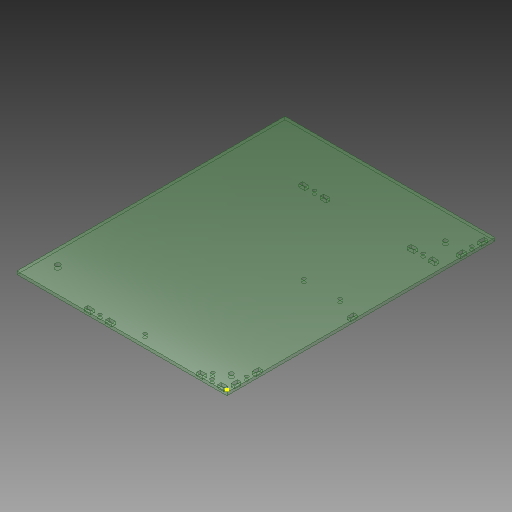
# Autodesk Inventor part: EE Base
Saved by Autodesk Inventor 2017 (Build 210142000, 142)
## iProperties
Created: 2016-07-27
Part Number: EE Base
Material: Polycarbonate, Green
Document SubType Name: Modeling
Designer: User
Density: 1.2 g/cm^3
Appearance: Polycarbonate - Clear(2)
Author: User
Autodesk Inventor part; units mm, degrees
(part 1 of 2)
ref_plane "YZ Plane" through (0, 0, 0) normal (1, 0, 0) x (0, 1, 0)
ref_plane "XZ Plane" through (0, 0, 0) normal (0, 1, 0) x (-1, 0, 0)
ref_plane "XY Plane" through (0, 0, 0) normal (0, 0, 1) x (1, 0, 0)
sketch "Sketch1" plane through (0, 0, 0) normal (0, 1, 0) x (-1, 0, 0)
  line L0 (-2.2365, 1.8101) -> (-2.2365, -264.9073)
  line L1 (-2.2365, -264.9073) -> (206.7635, -264.9073)
  line L2 (206.7635, -264.9073) -> (206.7635, 1.8101)
  line L3 (206.7635, 1.8101) -> (-2.2365, 1.8101)
  line L4 (58.9938, -133.7673) -> (58.8239, -133.3573)
  line L5 (58.8239, -133.3573) -> (58.5538, -133.0053)
  line L6 (58.5538, -133.0053) -> (58.2017, -132.7351)
  line L7 (58.2017, -132.7351) -> (57.7917, -132.5653)
  line L8 (57.7917, -132.5653) -> (57.3517, -132.5073)
  line L9 (57.3517, -132.5073) -> (56.9117, -132.5653)
  line L10 (56.9117, -132.5653) -> (56.5017, -132.7351)
  line L11 (56.5017, -132.7351) -> (56.1496, -133.0053)
  line L12 (56.1496, -133.0053) -> (55.8794, -133.3573)
  line L13 (55.8794, -133.3573) -> (55.7096, -133.7673)
  line L14 (55.7096, -133.7673) -> (55.6517, -134.2073)
  line L15 (55.6517, -134.2073) -> (55.7096, -134.6473)
  line L16 (55.7096, -134.6473) -> (55.8794, -135.0573)
  line L17 (55.8794, -135.0573) -> (56.1496, -135.4094)
  line L18 (56.1496, -135.4094) -> (56.5017, -135.6796)
  line L19 (56.5017, -135.6796) -> (56.9117, -135.8494)
  line L20 (56.9117, -135.8494) -> (57.3517, -135.9073)
  line L21 (57.3517, -135.9073) -> (57.7917, -135.8494)
  line L22 (57.7917, -135.8494) -> (58.2017, -135.6796)
  line L23 (58.2017, -135.6796) -> (58.5538, -135.4094)
  line L24 (58.5538, -135.4094) -> (58.8239, -135.0573)
  line L25 (58.8239, -135.0573) -> (58.9938, -134.6473)
  line L26 (58.9938, -134.6473) -> (59.0517, -134.2073)
  line L27 (59.0517, -134.2073) -> (58.9938, -133.7673)
  line L28 (21.4352, -215.2075) -> (21.3112, -214.8261)
  line L29 (21.3112, -214.8261) -> (21.0963, -214.4874)
  line L30 (21.0963, -214.4874) -> (20.8039, -214.2129)
  line L31 (20.8039, -214.2129) -> (20.4525, -214.0196)
  line L32 (20.4525, -214.0196) -> (20.064, -213.9199)
  line L33 (20.064, -213.9199) -> (19.663, -213.9199)
  line L34 (19.663, -213.9199) -> (19.2745, -214.0196)
  line L35 (19.2745, -214.0196) -> (18.923, -214.2129)
  line L36 (18.923, -214.2129) -> (18.6307, -214.4874)
  line L37 (18.6307, -214.4874) -> (18.4157, -214.8261)
  line L38 (18.4157, -214.8261) -> (18.2918, -215.2075)
  line L39 (18.2918, -215.2075) -> (18.2666, -215.6077)
  line L40 (18.2666, -215.6077) -> (18.3418, -216.0017)
  line L41 (18.3418, -216.0017) -> (18.5126, -216.3646)
  line L42 (18.5126, -216.3646) -> (18.7682, -216.6737)
  line L43 (18.7682, -216.6737) -> (19.0927, -216.9094)
  line L44 (19.0927, -216.9094) -> (19.4656, -217.057)
  line L45 (19.4656, -217.057) -> (19.8635, -217.1073)
  line L46 (19.8635, -217.1073) -> (20.2614, -217.057)
  line L47 (20.2614, -217.057) -> (20.6343, -216.9094)
  line L48 (20.6343, -216.9094) -> (20.9587, -216.6737)
  line L49 (20.9587, -216.6737) -> (21.2144, -216.3646)
  line L50 (21.2144, -216.3646) -> (21.3852, -216.0017)
  line L51 (21.3852, -216.0017) -> (21.42, -215.8311)
  line L52 (21.42, -215.8311) -> (21.4247, -215.8041)
  line L53 (21.4247, -215.8041) -> (21.4604, -215.6077)
  line L54 (21.4604, -215.6077) -> (21.4352, -215.2075)
  line L55 (13.929, -15.8348) -> (13.7092, -15.3042)
  line L56 (13.7092, -15.3042) -> (13.3596, -14.8486)
  line L57 (13.3596, -14.8486) -> (12.904, -14.499)
  line L58 (12.904, -14.499) -> (12.3734, -14.2792)
  line L59 (12.3734, -14.2792) -> (11.804, -14.2042)
  line L60 (11.804, -14.2042) -> (11.2346, -14.2792)
  line L61 (11.2346, -14.2792) -> (10.704, -14.499)
  line L62 (10.704, -14.499) -> (10.2483, -14.8486)
  line L63 (10.2483, -14.8486) -> (9.8987, -15.3042)
  line L64 (9.8987, -15.3042) -> (9.679, -15.8348)
  line L65 (9.679, -15.8348) -> (9.604, -16.4042)
  line L66 (9.604, -16.4042) -> (9.679, -16.9736)
  line L67 (9.679, -16.9736) -> (9.8987, -17.5042)
  line L68 (9.8987, -17.5042) -> (10.2483, -17.9599)
  line L69 (10.2483, -17.9599) -> (10.704, -18.3095)
  line L70 (10.704, -18.3095) -> (11.2346, -18.5293)
  line L71 (11.2346, -18.5293) -> (11.804, -18.6042)
  line L72 (11.804, -18.6042) -> (12.3734, -18.5293)
  line L73 (12.3734, -18.5293) -> (12.904, -18.3095)
  line L74 (12.904, -18.3095) -> (13.3596, -17.9599)
  line L75 (13.3596, -17.9599) -> (13.7092, -17.5042)
  line L76 (13.7092, -17.5042) -> (13.929, -16.9736)
  line L77 (13.929, -16.9736) -> (14.004, -16.4042)
  line L78 (14.004, -16.4042) -> (13.929, -15.8348)
  line L79 (2.7635, -0.1899) -> (2.7635, -3.7899)
  line L80 (2.7635, -3.7899) -> (8.9635, -3.7899)
  line L81 (8.9635, -3.7899) -> (8.9635, -0.1899)
  line L82 (8.9635, -0.1899) -> (2.7635, -0.1899)
  line L83 (3.1511, -245.3183) -> (2.9579, -244.9669)
  line L84 (2.9579, -244.9669) -> (2.6834, -244.6745)
  line L85 (2.6834, -244.6745) -> (2.3447, -244.4596)
  line L86 (2.3447, -244.4596) -> (1.9633, -244.3357)
  line L87 (1.9633, -244.3357) -> (1.5631, -244.3105)
  line L88 (1.5631, -244.3105) -> (1.1691, -244.3856)
  line L89 (1.1691, -244.3856) -> (0.8062, -244.5564)
  line L90 (0.8062, -244.5564) -> (0.4971, -244.812)
  line L91 (0.4971, -244.812) -> (0.2614, -245.1365)
  line L92 (0.2614, -245.1365) -> (0.1138, -245.5095)
  line L93 (0.1138, -245.5095) -> (0.0635, -245.9073)
  line L94 (0.0635, -245.9073) -> (0.1138, -246.3052)
  line L95 (0.1138, -246.3052) -> (0.2614, -246.6782)
  line L96 (0.2614, -246.6782) -> (0.4971, -247.0026)
  line L97 (0.4971, -247.0026) -> (0.8062, -247.2583)
  line L98 (0.8062, -247.2583) -> (1.1691, -247.429)
  line L99 (1.1691, -247.429) -> (1.5631, -247.5042)
  line L100 (1.5631, -247.5042) -> (1.9633, -247.479)
  line L101 (1.9633, -247.479) -> (2.3447, -247.3551)
  line L102 (2.3447, -247.3551) -> (2.6834, -247.1402)
  line L103 (2.6834, -247.1402) -> (2.9579, -246.8478)
  line L104 (2.9579, -246.8478) -> (3.1511, -246.4963)
  line L105 (3.1511, -246.4963) -> (3.2509, -246.1079)
  line L106 (3.2509, -246.1079) -> (3.2509, -245.7068)
  line L107 (3.2509, -245.7068) -> (3.1511, -245.3183)
  line L108 (-0.2365, -232.2073) -> (-0.2365, -238.4073)
  line L109 (-0.2365, -238.4073) -> (3.3635, -238.4073)
  line L110 (3.3635, -238.4073) -> (3.3635, -232.2073)
  line L111 (3.3635, -232.2073) -> (-0.2365, -232.2073)
  line L112 (-0.2365, -123.4758) -> (-0.2365, -129.7758)
  line L113 (-0.2365, -129.7758) -> (3.3635, -129.7758)
  line L114 (3.3635, -129.7758) -> (3.3635, -123.4758)
  line L115 (3.3635, -123.4758) -> (-0.2365, -123.4758)
  line L116 (3.1511, -21.0183) -> (2.9579, -20.6669)
  line L117 (2.9579, -20.6669) -> (2.6834, -20.3745)
  line L118 (2.6834, -20.3745) -> (2.3447, -20.1596)
  line L119 (2.3447, -20.1596) -> (1.9633, -20.0357)
  line L120 (1.9633, -20.0357) -> (1.5631, -20.0105)
  line L121 (1.5631, -20.0105) -> (1.1691, -20.0856)
  line L122 (1.1691, -20.0856) -> (0.8062, -20.2564)
  line L123 (0.8062, -20.2564) -> (0.4971, -20.5121)
  line L124 (0.4971, -20.5121) -> (0.2614, -20.8365)
  line L125 (0.2614, -20.8365) -> (0.1138, -21.2095)
  line L126 (0.1138, -21.2095) -> (0.0635, -21.6073)
  line L127 (0.0635, -21.6073) -> (0.1138, -22.0052)
  line L128 (0.1138, -22.0052) -> (0.2614, -22.3781)
  line L129 (0.2614, -22.3781) -> (0.4971, -22.7026)
  line L130 (0.4971, -22.7026) -> (0.8062, -22.9582)
  line L131 (0.8062, -22.9582) -> (1.1691, -23.129)
  line L132 (1.1691, -23.129) -> (1.5631, -23.2042)
  line L133 (1.5631, -23.2042) -> (1.9633, -23.179)
  line L134 (1.9633, -23.179) -> (2.3447, -23.0551)
  line L135 (2.3447, -23.0551) -> (2.6834, -22.8401)
  line L136 (2.6834, -22.8401) -> (2.9579, -22.5478)
  line L137 (2.9579, -22.5478) -> (3.1511, -22.1963)
  line L138 (3.1511, -22.1963) -> (3.2509, -21.8078)
  line L139 (3.2509, -21.8078) -> (3.2509, -21.4068)
  line L140 (3.2509, -21.4068) -> (3.1511, -21.0183)
  line L141 (6.1635, -213.6073) -> (6.1635, -217.2073)
  line L142 (6.1635, -217.2073) -> (12.3635, -217.2073)
  line L143 (12.3635, -217.2073) -> (12.3635, -213.6073)
  line L144 (12.3635, -213.6073) -> (6.1635, -213.6073)
  line L145 (-0.2365, -7.9073) -> (-0.2365, -14.1073)
  line L146 (-0.2365, -14.1073) -> (3.3635, -14.1073)
  line L147 (3.3635, -14.1073) -> (3.3635, -7.9073)
  line L148 (3.3635, -7.9073) -> (-0.2365, -7.9073)
  line L149 (-0.2365, -253.4073) -> (-0.2365, -259.6074)
  line L150 (-0.2365, -259.6074) -> (3.3635, -259.6074)
  line L151 (3.3635, -259.6074) -> (3.3635, -253.4073)
  line L152 (3.3635, -253.4073) -> (-0.2365, -253.4073)
  line L153 (-0.2365, -29.1073) -> (-0.2365, -35.3073)
  line L154 (-0.2365, -35.3073) -> (3.3635, -35.3073)
  line L155 (3.3635, -35.3073) -> (3.3635, -29.1073)
  line L156 (3.3635, -29.1073) -> (-0.2365, -29.1073)
  line L157 (18.0352, -1.7901) -> (17.9112, -1.4087)
  line L158 (17.9112, -1.4087) -> (17.6963, -1.07)
  line L159 (17.6963, -1.07) -> (17.4039, -0.7955)
  line L160 (17.4039, -0.7955) -> (17.0525, -0.6023)
  line L161 (17.0525, -0.6023) -> (16.664, -0.5025)
  line L162 (16.664, -0.5025) -> (16.263, -0.5025)
  line L163 (16.263, -0.5025) -> (15.8745, -0.6023)
  line L164 (15.8745, -0.6023) -> (15.523, -0.7955)
  line L165 (15.523, -0.7955) -> (15.2307, -1.07)
  line L166 (15.2307, -1.07) -> (15.0158, -1.4087)
  line L167 (15.0158, -1.4087) -> (14.8918, -1.7901)
  line L168 (14.8918, -1.7901) -> (14.8667, -2.1903)
  line L169 (14.8667, -2.1903) -> (14.9418, -2.5843)
  line L170 (14.9418, -2.5843) -> (15.1126, -2.9472)
  line L171 (15.1126, -2.9472) -> (15.3682, -3.2563)
  line L172 (15.3682, -3.2563) -> (15.6927, -3.492)
  line L173 (15.6927, -3.492) -> (16.0656, -3.6396)
  line L174 (16.0656, -3.6396) -> (16.4635, -3.6899)
  line L175 (16.4635, -3.6899) -> (16.8614, -3.6396)
  line L176 (16.8614, -3.6396) -> (17.2343, -3.492)
  line L177 (17.2343, -3.492) -> (17.5587, -3.2563)
  line L178 (17.5587, -3.2563) -> (17.8144, -2.9472)
  line L179 (17.8144, -2.9472) -> (17.9852, -2.5843)
  line L180 (17.9852, -2.5843) -> (18.0604, -2.1903)
  line L181 (18.0604, -2.1903) -> (18.0352, -1.7901)
  line L182 (23.4056, -7.4674) -> (23.2357, -7.0573)
  line L183 (23.2357, -7.0573) -> (22.9656, -6.7052)
  line L184 (22.9656, -6.7052) -> (22.6135, -6.4351)
  line L185 (22.6135, -6.4351) -> (22.2035, -6.2653)
  line L186 (22.2035, -6.2653) -> (21.7635, -6.2073)
  line L187 (21.7635, -6.2073) -> (21.3235, -6.2653)
  line L188 (21.3235, -6.2653) -> (20.9135, -6.4351)
  line L189 (20.9135, -6.4351) -> (20.5614, -6.7052)
  line L190 (20.5614, -6.7052) -> (20.2912, -7.0573)
  line L191 (20.2912, -7.0573) -> (20.1214, -7.4674)
  line L192 (20.1214, -7.4674) -> (20.0635, -7.9073)
  line L193 (20.0635, -7.9073) -> (20.1214, -8.3473)
  line L194 (20.1214, -8.3473) -> (20.2912, -8.7573)
  line L195 (20.2912, -8.7573) -> (20.5614, -9.1094)
  line L196 (20.5614, -9.1094) -> (20.9135, -9.3796)
  line L197 (20.9135, -9.3796) -> (21.3235, -9.5494)
  line L198 (21.3235, -9.5494) -> (21.7635, -9.6073)
  line L199 (21.7635, -9.6073) -> (22.2035, -9.5494)
  line L200 (22.2035, -9.5494) -> (22.6135, -9.3796)
  line L201 (22.6135, -9.3796) -> (22.9656, -9.1094)
  line L202 (22.9656, -9.1094) -> (23.2357, -8.7573)
  line L203 (23.2357, -8.7573) -> (23.4056, -8.3473)
  line L204 (23.4056, -8.3473) -> (23.4635, -7.9073)
  line L205 (23.4635, -7.9073) -> (23.4056, -7.4674)
  line L206 (23.7088, -134.5768) -> (23.539, -134.1668)
  line L207 (23.539, -134.1668) -> (23.2688, -133.8147)
  line L208 (23.2688, -133.8147) -> (22.9168, -133.5446)
  line L209 (22.9168, -133.5446) -> (22.5068, -133.3747)
  line L210 (22.5068, -133.3747) -> (22.0667, -133.3168)
  line L211 (22.0667, -133.3168) -> (21.6268, -133.3747)
  line L212 (21.6268, -133.3747) -> (21.2168, -133.5446)
  line L213 (21.2168, -133.5446) -> (20.8647, -133.8147)
  line L214 (20.8647, -133.8147) -> (20.5945, -134.1668)
  line L215 (20.5945, -134.1668) -> (20.4247, -134.5768)
  line L216 (20.4247, -134.5768) -> (20.3668, -135.0168)
  line L217 (20.3668, -135.0168) -> (20.4247, -135.4568)
  line L218 (20.4247, -135.4568) -> (20.5945, -135.8668)
  line L219 (20.5945, -135.8668) -> (20.8647, -136.2189)
  line L220 (20.8647, -136.2189) -> (21.2168, -136.489)
  line L221 (21.2168, -136.489) -> (21.6268, -136.6589)
  line L222 (21.6268, -136.6589) -> (22.0667, -136.7168)
  line L223 (22.0667, -136.7168) -> (22.5068, -136.6589)
  line L224 (22.5068, -136.6589) -> (22.9168, -136.489)
  line L225 (22.9168, -136.489) -> (23.2688, -136.2189)
  line L226 (23.2688, -136.2189) -> (23.539, -135.8668)
  line L227 (23.539, -135.8668) -> (23.7088, -135.4568)
  line L228 (23.7088, -135.4568) -> (23.7667, -135.0168)
  line L229 (23.7667, -135.0168) -> (23.7088, -134.5768)
  line L230 (27.3634, -213.6073) -> (27.3634, -217.2073)
  line L231 (27.3634, -217.2073) -> (33.5635, -217.2073)
  line L232 (33.5635, -217.2073) -> (33.5635, -213.6073)
  line L233 (33.5635, -213.6073) -> (27.3634, -213.6073)
  line L234 (23.9635, -0.1899) -> (23.9635, -3.7899)
  line L235 (23.9635, -3.7899) -> (30.1635, -3.7899)
  line L236 (30.1635, -3.7899) -> (30.1635, -0.1899)
  line L237 (30.1635, -0.1899) -> (23.9635, -0.1899)
  line L238 (90.6056, -7.461) -> (90.4357, -7.051)
  line L239 (90.4357, -7.051) -> (90.1656, -6.6989)
  line L240 (90.1656, -6.6989) -> (89.8135, -6.4288)
  line L241 (89.8135, -6.4288) -> (89.4035, -6.2589)
  line L242 (89.4035, -6.2589) -> (88.9635, -6.201)
  line L243 (88.9635, -6.201) -> (88.5235, -6.2589)
  line L244 (88.5235, -6.2589) -> (88.1135, -6.4288)
  line L245 (88.1135, -6.4288) -> (87.7614, -6.6989)
  line L246 (87.7614, -6.6989) -> (87.4913, -7.051)
  line L247 (87.4913, -7.051) -> (87.3214, -7.461)
  line L248 (87.3214, -7.461) -> (87.2635, -7.901)
  line L249 (87.2635, -7.901) -> (87.3214, -8.341)
  line L250 (87.3214, -8.341) -> (87.4913, -8.751)
  line L251 (87.4913, -8.751) -> (87.7614, -9.1031)
  line L252 (87.7614, -9.1031) -> (88.1135, -9.3733)
  line L253 (88.1135, -9.3733) -> (88.5235, -9.5431)
  line L254 (88.5235, -9.5431) -> (88.9635, -9.601)
  line L255 (88.9635, -9.601) -> (89.4035, -9.5431)
  line L256 (89.4035, -9.5431) -> (89.8135, -9.3733)
  line L257 (89.8135, -9.3733) -> (90.1656, -9.1031)
  line L258 (90.1656, -9.1031) -> (90.4357, -8.751)
  line L259 (90.4357, -8.751) -> (90.6056, -8.341)
  line L260 (90.6056, -8.341) -> (90.6635, -7.901)
  line L261 (90.6635, -7.901) -> (90.6056, -7.461)
  line L262 (114.3635, -213.6073) -> (114.3635, -217.2073)
  line L263 (114.3635, -217.2073) -> (120.5635, -217.2073)
  line L264 (120.5635, -217.2073) -> (120.5635, -213.6073)
  line L265 (120.5635, -213.6073) -> (114.3635, -213.6073)
  line L266 (129.6352, -215.2075) -> (129.5112, -214.8261)
  line L267 (129.5112, -214.8261) -> (129.2963, -214.4874)
  line L268 (129.2963, -214.4874) -> (129.0039, -214.2129)
  line L269 (129.0039, -214.2129) -> (128.6525, -214.0196)
  line L270 (128.6525, -214.0196) -> (128.264, -213.9199)
  line L271 (128.264, -213.9199) -> (127.863, -213.9199)
  line L272 (127.863, -213.9199) -> (127.4745, -214.0196)
  line L273 (127.4745, -214.0196) -> (127.123, -214.2129)
  line L274 (127.123, -214.2129) -> (126.8307, -214.4874)
  line L275 (126.8307, -214.4874) -> (126.6158, -214.8261)
  line L276 (126.6158, -214.8261) -> (126.4918, -215.2075)
  line L277 (126.4918, -215.2075) -> (126.4666, -215.6077)
  line L278 (126.4666, -215.6077) -> (126.5418, -216.0017)
  line L279 (126.5418, -216.0017) -> (126.7125, -216.3646)
  line L280 (126.7125, -216.3646) -> (126.9682, -216.6737)
  line L281 (126.9682, -216.6737) -> (127.2927, -216.9094)
  line L282 (127.2927, -216.9094) -> (127.6656, -217.057)
  line L283 (127.6656, -217.057) -> (128.0635, -217.1073)
  line L284 (128.0635, -217.1073) -> (128.4614, -217.057)
  line L285 (128.4614, -217.057) -> (128.8343, -216.9094)
  line L286 (128.8343, -216.9094) -> (129.1588, -216.6737)
  line L287 (129.1588, -216.6737) -> (129.4144, -216.3646)
  line L288 (129.4144, -216.3646) -> (129.5852, -216.0017)
  line L289 (129.5852, -216.0017) -> (129.6603, -215.6077)
  line L290 (129.6603, -215.6077) -> (129.6352, -215.2075)
  line L291 (194.4204, -23.2582) -> (194.1699, -22.6533)
  line L292 (194.1699, -22.6533) -> (193.7713, -22.1339)
  line L293 (193.7713, -22.1339) -> (193.2519, -21.7353)
  line L294 (193.2519, -21.7353) -> (192.647, -21.4848)
  line L295 (192.647, -21.4848) -> (191.9979, -21.3993)
  line L296 (191.9979, -21.3993) -> (191.3488, -21.4848)
  line L297 (191.3488, -21.4848) -> (190.7439, -21.7353)
  line L298 (190.7439, -21.7353) -> (190.2245, -22.1339)
  line L299 (190.2245, -22.1339) -> (189.8259, -22.6533)
  line L300 (189.8259, -22.6533) -> (189.5754, -23.2582)
  line L301 (189.5754, -23.2582) -> (189.4899, -23.9073)
  line L302 (189.4899, -23.9073) -> (189.5754, -24.5564)
  line L303 (189.5754, -24.5564) -> (189.8259, -25.1613)
  line L304 (189.8259, -25.1613) -> (190.2245, -25.6807)
  line L305 (190.2245, -25.6807) -> (190.7439, -26.0793)
  line L306 (190.7439, -26.0793) -> (191.3488, -26.3299)
  line L307 (191.3488, -26.3299) -> (191.9979, -26.4153)
  line L308 (191.9979, -26.4153) -> (192.647, -26.3299)
  line L309 (192.647, -26.3299) -> (193.2519, -26.0793)
  line L310 (193.2519, -26.0793) -> (193.7713, -25.6807)
  line L311 (193.7713, -25.6807) -> (194.1699, -25.1613)
  line L312 (194.1699, -25.1613) -> (194.4204, -24.5564)
  line L313 (194.4204, -24.5564) -> (194.5059, -23.9073)
  line L314 (194.5059, -23.9073) -> (194.4204, -23.2582)
  line L315 (135.5635, -213.6073) -> (135.5635, -217.2073)
  line L316 (135.5635, -217.2073) -> (141.7635, -217.2073)
  line L317 (141.7635, -217.2073) -> (141.7635, -213.6073)
  line L318 (141.7635, -213.6073) -> (135.5635, -213.6073)
  line L319 (135.5635, -0.1899) -> (135.5635, -3.7899)
  line L320 (135.5635, -3.7899) -> (141.7635, -3.7899)
  line L321 (141.7635, -3.7899) -> (141.7635, -0.1899)
  line L322 (141.7635, -0.1899) -> (135.5635, -0.1899)
  line L323 (114.3635, -0.1899) -> (114.3635, -3.7899)
  line L324 (114.3635, -3.7899) -> (120.5635, -3.7899)
  line L325 (120.5635, -3.7899) -> (120.5635, -0.1899)
  line L326 (120.5635, -0.1899) -> (114.3635, -0.1899)
  line L327 (129.6352, -1.7901) -> (129.5112, -1.4087)
  line L328 (129.5112, -1.4087) -> (129.2963, -1.07)
  line L329 (129.2963, -1.07) -> (129.0039, -0.7955)
  line L330 (129.0039, -0.7955) -> (128.6525, -0.6023)
  line L331 (128.6525, -0.6023) -> (128.264, -0.5025)
  line L332 (128.264, -0.5025) -> (127.863, -0.5025)
  line L333 (127.863, -0.5025) -> (127.4745, -0.6023)
  line L334 (127.4745, -0.6023) -> (127.123, -0.7955)
  line L335 (127.123, -0.7955) -> (126.8307, -1.07)
  line L336 (126.8307, -1.07) -> (126.6158, -1.4087)
  line L337 (126.6158, -1.4087) -> (126.4918, -1.7901)
  line L338 (126.4918, -1.7901) -> (126.4666, -2.1903)
  line L339 (126.4666, -2.1903) -> (126.5418, -2.5843)
  line L340 (126.5418, -2.5843) -> (126.7125, -2.9472)
  line L341 (126.7125, -2.9472) -> (126.9682, -3.2563)
  line L342 (126.9682, -3.2563) -> (127.2927, -3.492)
  line L343 (127.2927, -3.492) -> (127.6656, -3.6396)
  line L344 (127.6656, -3.6396) -> (128.0635, -3.6899)
  line L345 (128.0635, -3.6899) -> (128.4614, -3.6396)
  line L346 (128.4614, -3.6396) -> (128.8343, -3.492)
  line L347 (128.8343, -3.492) -> (129.1588, -3.2563)
  line L348 (129.1588, -3.2563) -> (129.4144, -2.9472)
  line L349 (129.4144, -2.9472) -> (129.5852, -2.5843)
  line L350 (129.5852, -2.5843) -> (129.6603, -2.1903)
  line L351 (129.6603, -2.1903) -> (129.6352, -1.7901)
  line L352 (21.8831, -237.0851) -> (21.685, -236.5461)
  line L353 (21.685, -236.5461) -> (21.354, -236.0767)
  line L354 (21.354, -236.0767) -> (20.9129, -235.7089)
  line L355 (20.9129, -235.7089) -> (20.3916, -235.4679)
  line L356 (20.3916, -235.4679) -> (19.8257, -235.37)
  line L357 (19.8257, -235.37) -> (19.2537, -235.4219)
  line L358 (19.2537, -235.4219) -> (18.7147, -235.6201)
  line L359 (18.7147, -235.6201) -> (18.2453, -235.951)
  line L360 (18.2453, -235.951) -> (17.8776, -236.3922)
  line L361 (17.8776, -236.3922) -> (17.6365, -236.9134)
  line L362 (17.6365, -236.9134) -> (17.5386, -237.4793)
  line L363 (17.5386, -237.4793) -> (17.5905, -238.0513)
  line L364 (17.5905, -238.0513) -> (17.7887, -238.5903)
  line L365 (17.7887, -238.5903) -> (18.1196, -239.0597)
  line L366 (18.1196, -239.0597) -> (18.5608, -239.4274)
  line L367 (18.5608, -239.4274) -> (19.0821, -239.6685)
  line L368 (19.0821, -239.6685) -> (19.648, -239.7664)
  line L369 (19.648, -239.7664) -> (20.22, -239.7145)
  line L370 (20.22, -239.7145) -> (20.759, -239.5163)
  line L371 (20.759, -239.5163) -> (21.2284, -239.1854)
  line L372 (21.2284, -239.1854) -> (21.5961, -238.7443)
  line L373 (21.5961, -238.7443) -> (21.8371, -238.223)
  line L374 (21.8371, -238.223) -> (21.9351, -237.6571)
  line L375 (21.9351, -237.6571) -> (21.8831, -237.0851)
  point P0 (0, 0)
  constraints: 752 end point
extrude "Extrusion1" add sketch "Sketch1" along normal blind 3
sketch "Sketch2" plane through (0, 3, 0) normal (0, 1, 0) x (1, 0, 0)
  line L0 (0.2365, 123.4758) -> (-3.3635, 123.4758) projected
  line L1 (-3.3635, 123.4758) -> (-3.3635, 129.7758) projected
  line L2 (-3.3635, 129.7758) -> (0.2365, 129.7758) projected
  line L3 (0.2365, 129.7758) -> (0.2365, 123.4758) projected
  line L4 (-23.9635, 0.1899) -> (-30.1635, 0.1899) projected
  line L5 (-30.1635, 0.1899) -> (-30.1635, 3.7899) projected
  line L6 (-30.1635, 3.7899) -> (-23.9635, 3.7899) projected
  line L7 (-23.9635, 3.7899) -> (-23.9635, 0.1899) projected
  line L8 (-27.3634, 213.6073) -> (-33.5635, 213.6073) projected
  line L9 (-33.5635, 213.6073) -> (-33.5635, 217.2073) projected
  line L10 (-33.5635, 217.2073) -> (-27.3634, 217.2073) projected
  line L11 (-27.3634, 217.2073) -> (-27.3634, 213.6073) projected
  line L12 (-135.5635, 0.1899) -> (-141.7635, 0.1899) projected
  line L13 (-141.7635, 0.1899) -> (-141.7635, 3.7899) projected
  line L14 (-141.7635, 3.7899) -> (-135.5635, 3.7899) projected
  line L15 (-135.5635, 3.7899) -> (-135.5635, 0.1899) projected
  line L16 (-135.5635, 213.6073) -> (-141.7635, 213.6073) projected
  line L17 (-141.7635, 213.6073) -> (-141.7635, 217.2073) projected
  line L18 (-141.7635, 217.2073) -> (-135.5635, 217.2073) projected
  line L19 (-135.5635, 217.2073) -> (-135.5635, 213.6073) projected
  line L20 (0.2365, 29.1073) -> (-3.3635, 29.1073) projected
  line L21 (-3.3635, 29.1073) -> (-3.3635, 35.3073) projected
  line L22 (-3.3635, 35.3073) -> (0.2365, 35.3073) projected
  line L23 (0.2365, 35.3073) -> (0.2365, 29.1073) projected
  line L24 (0.2365, 253.4073) -> (-3.3635, 253.4073) projected
  line L25 (-3.3635, 253.4073) -> (-3.3635, 259.6074) projected
  line L26 (-3.3635, 259.6074) -> (0.2365, 259.6074) projected
  line L27 (0.2365, 259.6074) -> (0.2365, 253.4073) projected
  line L28 (-114.3635, 0.1899) -> (-120.5635, 0.1899) projected
  line L29 (-120.5635, 0.1899) -> (-120.5635, 3.7899) projected
  line L30 (-120.5635, 3.7899) -> (-114.3635, 3.7899) projected
  line L31 (-114.3635, 3.7899) -> (-114.3635, 0.1899) projected
  line L32 (-114.3635, 213.6073) -> (-120.5635, 213.6073) projected
  line L33 (-120.5635, 213.6073) -> (-120.5635, 217.2073) projected
  line L34 (-120.5635, 217.2073) -> (-114.3635, 217.2073) projected
  line L35 (-114.3635, 217.2073) -> (-114.3635, 213.6073) projected
  line L36 (0.2365, 232.2073) -> (-3.3635, 232.2073) projected
  line L37 (-3.3635, 232.2073) -> (-3.3635, 238.4073) projected
  line L38 (-3.3635, 238.4073) -> (0.2365, 238.4073) projected
  line L39 (0.2365, 238.4073) -> (0.2365, 232.2073) projected
  line L40 (-2.7635, 0.1899) -> (-8.9635, 0.1899) projected
  line L41 (-8.9635, 0.1899) -> (-8.9635, 3.7899) projected
  line L42 (-8.9635, 3.7899) -> (-2.7635, 3.7899) projected
  line L43 (-2.7635, 3.7899) -> (-2.7635, 0.1899) projected
  line L44 (0.2365, 7.9073) -> (-3.3635, 7.9073) projected
  line L45 (-3.3635, 7.9073) -> (-3.3635, 14.1073) projected
  line L46 (-3.3635, 14.1073) -> (0.2365, 14.1073) projected
  line L47 (0.2365, 14.1073) -> (0.2365, 7.9073) projected
  line L48 (-6.1635, 213.6073) -> (-12.3635, 213.6073) projected
  line L49 (-12.3635, 213.6073) -> (-12.3635, 217.2073) projected
  line L50 (-12.3635, 217.2073) -> (-6.1635, 217.2073) projected
  line L51 (-6.1635, 217.2073) -> (-6.1635, 213.6073) projected
  line L52 (-194.4204, 23.2582) -> (-194.5059, 23.9073) projected
  line L53 (-194.5059, 23.9073) -> (-194.4204, 24.5564) projected
  line L54 (-194.4204, 24.5564) -> (-194.1699, 25.1613) projected
  line L55 (-194.1699, 25.1613) -> (-193.7713, 25.6807) projected
  line L56 (-193.7713, 25.6807) -> (-193.2519, 26.0793) projected
  line L57 (-193.2519, 26.0793) -> (-192.647, 26.3299) projected
  line L58 (-192.647, 26.3299) -> (-191.9979, 26.4153) projected
  line L59 (-191.9979, 26.4153) -> (-191.3488, 26.3299) projected
  line L60 (-191.3488, 26.3299) -> (-190.7439, 26.0793) projected
  line L61 (-190.7439, 26.0793) -> (-190.2245, 25.6807) projected
  line L62 (-190.2245, 25.6807) -> (-189.8259, 25.1613) projected
  line L63 (-189.8259, 25.1613) -> (-189.5754, 24.5564) projected
  line L64 (-189.5754, 24.5564) -> (-189.4899, 23.9073) projected
  line L65 (-189.4899, 23.9073) -> (-189.5754, 23.2582) projected
  line L66 (-189.5754, 23.2582) -> (-189.8259, 22.6533) projected
  line L67 (-189.8259, 22.6533) -> (-190.2245, 22.1339) projected
  line L68 (-190.2245, 22.1339) -> (-190.7439, 21.7353) projected
  line L69 (-190.7439, 21.7353) -> (-191.3488, 21.4848) projected
  line L70 (-191.3488, 21.4848) -> (-191.9979, 21.3993) projected
  line L71 (-191.9979, 21.3993) -> (-192.647, 21.4848) projected
  line L72 (-192.647, 21.4848) -> (-193.2519, 21.7353) projected
  line L73 (-193.2519, 21.7353) -> (-193.7713, 22.1339) projected
  line L74 (-193.7713, 22.1339) -> (-194.1699, 22.6533) projected
  line L75 (-194.1699, 22.6533) -> (-194.4204, 23.2582) projected
  line L76 (-13.929, 15.8348) -> (-14.004, 16.4042) projected
  line L77 (-14.004, 16.4042) -> (-13.929, 16.9736) projected
  line L78 (-13.929, 16.9736) -> (-13.7092, 17.5042) projected
  line L79 (-13.7092, 17.5042) -> (-13.3596, 17.9599) projected
  line L80 (-13.3596, 17.9599) -> (-12.904, 18.3095) projected
  line L81 (-12.904, 18.3095) -> (-12.3734, 18.5293) projected
  line L82 (-12.3734, 18.5293) -> (-11.804, 18.6042) projected
  line L83 (-11.804, 18.6042) -> (-11.2346, 18.5293) projected
  line L84 (-11.2346, 18.5293) -> (-10.704, 18.3095) projected
  line L85 (-10.704, 18.3095) -> (-10.2483, 17.9599) projected
  line L86 (-10.2483, 17.9599) -> (-9.8987, 17.5042) projected
  line L87 (-9.8987, 17.5042) -> (-9.679, 16.9736) projected
  line L88 (-9.679, 16.9736) -> (-9.604, 16.4042) projected
  line L89 (-9.604, 16.4042) -> (-9.679, 15.8348) projected
  line L90 (-9.679, 15.8348) -> (-9.8987, 15.3042) projected
  line L91 (-9.8987, 15.3042) -> (-10.2483, 14.8486) projected
  line L92 (-10.2483, 14.8486) -> (-10.704, 14.499) projected
  line L93 (-10.704, 14.499) -> (-11.2346, 14.2792) projected
  line L94 (-11.2346, 14.2792) -> (-11.804, 14.2042) projected
  line L95 (-11.804, 14.2042) -> (-12.3734, 14.2792) projected
  line L96 (-12.3734, 14.2792) -> (-12.904, 14.499) projected
  line L97 (-12.904, 14.499) -> (-13.3596, 14.8486) projected
  line L98 (-13.3596, 14.8486) -> (-13.7092, 15.3042) projected
  line L99 (-13.7092, 15.3042) -> (-13.929, 15.8348) projected
  line L100 (-21.8831, 237.0851) -> (-21.9351, 237.6571) projected
  line L101 (-21.9351, 237.6571) -> (-21.8371, 238.223) projected
  line L102 (-21.8371, 238.223) -> (-21.5961, 238.7443) projected
  line L103 (-21.5961, 238.7443) -> (-21.2284, 239.1854) projected
  line L104 (-21.2284, 239.1854) -> (-20.759, 239.5163) projected
  line L105 (-20.759, 239.5163) -> (-20.22, 239.7145) projected
  line L106 (-20.22, 239.7145) -> (-19.648, 239.7664) projected
  line L107 (-19.648, 239.7664) -> (-19.0821, 239.6685) projected
  line L108 (-19.0821, 239.6685) -> (-18.5608, 239.4274) projected
  line L109 (-18.5608, 239.4274) -> (-18.1196, 239.0597) projected
  line L110 (-18.1196, 239.0597) -> (-17.7887, 238.5903) projected
  line L111 (-17.7887, 238.5903) -> (-17.5905, 238.0513) projected
  line L112 (-17.5905, 238.0513) -> (-17.5386, 237.4793) projected
  line L113 (-17.5386, 237.4793) -> (-17.6365, 236.9134) projected
  line L114 (-17.6365, 236.9134) -> (-17.8776, 236.3922) projected
  line L115 (-17.8776, 236.3922) -> (-18.2453, 235.951) projected
  line L116 (-18.2453, 235.951) -> (-18.7147, 235.6201) projected
  line L117 (-18.7147, 235.6201) -> (-19.2537, 235.4219) projected
  line L118 (-19.2537, 235.4219) -> (-19.8257, 235.37) projected
  line L119 (-19.8257, 235.37) -> (-20.3916, 235.4679) projected
  line L120 (-20.3916, 235.4679) -> (-20.9129, 235.7089) projected
  line L121 (-20.9129, 235.7089) -> (-21.354, 236.0767) projected
  line L122 (-21.354, 236.0767) -> (-21.685, 236.5461) projected
  line L123 (-21.685, 236.5461) -> (-21.8831, 237.0851) projected
  line L124 (-23.4056, 7.4674) -> (-23.4635, 7.9073) projected
  line L125 (-23.4635, 7.9073) -> (-23.4056, 8.3473) projected
  line L126 (-23.4056, 8.3473) -> (-23.2357, 8.7573) projected
  line L127 (-23.2357, 8.7573) -> (-22.9656, 9.1094) projected
  line L128 (-22.9656, 9.1094) -> (-22.6135, 9.3796) projected
  line L129 (-22.6135, 9.3796) -> (-22.2035, 9.5494) projected
  line L130 (-22.2035, 9.5494) -> (-21.7635, 9.6073) projected
  line L131 (-21.7635, 9.6073) -> (-21.3235, 9.5494) projected
  line L132 (-21.3235, 9.5494) -> (-20.9135, 9.3796) projected
  line L133 (-20.9135, 9.3796) -> (-20.5614, 9.1094) projected
  line L134 (-20.5614, 9.1094) -> (-20.2912, 8.7573) projected
  line L135 (-20.2912, 8.7573) -> (-20.1214, 8.3473) projected
  line L136 (-20.1214, 8.3473) -> (-20.0635, 7.9073) projected
  line L137 (-20.0635, 7.9073) -> (-20.1214, 7.4674) projected
  line L138 (-20.1214, 7.4674) -> (-20.2912, 7.0573) projected
  line L139 (-20.2912, 7.0573) -> (-20.5614, 6.7052) projected
  line L140 (-20.5614, 6.7052) -> (-20.9135, 6.4351) projected
  line L141 (-20.9135, 6.4351) -> (-21.3235, 6.2653) projected
  line L142 (-21.3235, 6.2653) -> (-21.7635, 6.2073) projected
  line L143 (-21.7635, 6.2073) -> (-22.2035, 6.2653) projected
  line L144 (-22.2035, 6.2653) -> (-22.6135, 6.4351) projected
  line L145 (-22.6135, 6.4351) -> (-22.9656, 6.7052) projected
  line L146 (-22.9656, 6.7052) -> (-23.2357, 7.0573) projected
  line L147 (-23.2357, 7.0573) -> (-23.4056, 7.4674) projected
  line L148 (-58.9938, 133.7673) -> (-59.0517, 134.2073) projected
  line L149 (-59.0517, 134.2073) -> (-58.9938, 134.6473) projected
  line L150 (-58.9938, 134.6473) -> (-58.8239, 135.0573) projected
  line L151 (-58.8239, 135.0573) -> (-58.5538, 135.4094) projected
  line L152 (-58.5538, 135.4094) -> (-58.2017, 135.6796) projected
  line L153 (-58.2017, 135.6796) -> (-57.7917, 135.8494) projected
  line L154 (-57.7917, 135.8494) -> (-57.3517, 135.9073) projected
  line L155 (-57.3517, 135.9073) -> (-56.9117, 135.8494) projected
  line L156 (-56.9117, 135.8494) -> (-56.5017, 135.6796) projected
  line L157 (-56.5017, 135.6796) -> (-56.1496, 135.4094) projected
  line L158 (-56.1496, 135.4094) -> (-55.8794, 135.0573) projected
  line L159 (-55.8794, 135.0573) -> (-55.7096, 134.6473) projected
  line L160 (-55.7096, 134.6473) -> (-55.6517, 134.2073) projected
  line L161 (-55.6517, 134.2073) -> (-55.7096, 133.7673) projected
  line L162 (-55.7096, 133.7673) -> (-55.8794, 133.3573) projected
  line L163 (-55.8794, 133.3573) -> (-56.1496, 133.0053) projected
  line L164 (-56.1496, 133.0053) -> (-56.5017, 132.7351) projected
  line L165 (-56.5017, 132.7351) -> (-56.9117, 132.5653) projected
  line L166 (-56.9117, 132.5653) -> (-57.3517, 132.5073) projected
  line L167 (-57.3517, 132.5073) -> (-57.7917, 132.5653) projected
  line L168 (-57.7917, 132.5653) -> (-58.2017, 132.7351) projected
  line L169 (-58.2017, 132.7351) -> (-58.5538, 133.0053) projected
  line L170 (-58.5538, 133.0053) -> (-58.8239, 133.3573) projected
  line L171 (-58.8239, 133.3573) -> (-58.9938, 133.7673) projected
  line L172 (-90.6056, 7.461) -> (-90.6635, 7.901) projected
  line L173 (-90.6635, 7.901) -> (-90.6056, 8.341) projected
  line L174 (-90.6056, 8.341) -> (-90.4357, 8.751) projected
  line L175 (-90.4357, 8.751) -> (-90.1656, 9.1031) projected
  line L176 (-90.1656, 9.1031) -> (-89.8135, 9.3733) projected
  line L177 (-89.8135, 9.3733) -> (-89.4035, 9.5431) projected
  line L178 (-89.4035, 9.5431) -> (-88.9635, 9.601) projected
  line L179 (-88.9635, 9.601) -> (-88.5235, 9.5431) projected
  line L180 (-88.5235, 9.5431) -> (-88.1135, 9.3733) projected
  line L181 (-88.1135, 9.3733) -> (-87.7614, 9.1031) projected
  line L182 (-87.7614, 9.1031) -> (-87.4913, 8.751) projected
  line L183 (-87.4913, 8.751) -> (-87.3214, 8.341) projected
  line L184 (-87.3214, 8.341) -> (-87.2635, 7.901) projected
  line L185 (-87.2635, 7.901) -> (-87.3214, 7.461) projected
  line L186 (-87.3214, 7.461) -> (-87.4913, 7.051) projected
  line L187 (-87.4913, 7.051) -> (-87.7614, 6.6989) projected
  line L188 (-87.7614, 6.6989) -> (-88.1135, 6.4288) projected
  line L189 (-88.1135, 6.4288) -> (-88.5235, 6.2589) projected
  line L190 (-88.5235, 6.2589) -> (-88.9635, 6.201) projected
  line L191 (-88.9635, 6.201) -> (-89.4035, 6.2589) projected
  line L192 (-89.4035, 6.2589) -> (-89.8135, 6.4288) projected
  line L193 (-89.8135, 6.4288) -> (-90.1656, 6.6989) projected
  line L194 (-90.1656, 6.6989) -> (-90.4357, 7.051) projected
  line L195 (-90.4357, 7.051) -> (-90.6056, 7.461) projected
  line L196 (-23.7088, 134.5768) -> (-23.7667, 135.0168) projected
  line L197 (-23.7667, 135.0168) -> (-23.7088, 135.4568) projected
  line L198 (-23.7088, 135.4568) -> (-23.539, 135.8668) projected
  line L199 (-23.539, 135.8668) -> (-23.2688, 136.2189) projected
  line L200 (-23.2688, 136.2189) -> (-22.9168, 136.489) projected
  line L201 (-22.9168, 136.489) -> (-22.5068, 136.6589) projected
  line L202 (-22.5068, 136.6589) -> (-22.0667, 136.7168) projected
  line L203 (-22.0667, 136.7168) -> (-21.6268, 136.6589) projected
  line L204 (-21.6268, 136.6589) -> (-21.2168, 136.489) projected
  line L205 (-21.2168, 136.489) -> (-20.8647, 136.2189) projected
  line L206 (-20.8647, 136.2189) -> (-20.5945, 135.8668) projected
  line L207 (-20.5945, 135.8668) -> (-20.4247, 135.4568) projected
  line L208 (-20.4247, 135.4568) -> (-20.3668, 135.0168) projected
  line L209 (-20.3668, 135.0168) -> (-20.4247, 134.5768) projected
  line L210 (-20.4247, 134.5768) -> (-20.5945, 134.1668) projected
  line L211 (-20.5945, 134.1668) -> (-20.8647, 133.8147) projected
  line L212 (-20.8647, 133.8147) -> (-21.2168, 133.5446) projected
  line L213 (-21.2168, 133.5446) -> (-21.6268, 133.3747) projected
  line L214 (-21.6268, 133.3747) -> (-22.0667, 133.3168) projected
  line L215 (-22.0667, 133.3168) -> (-22.5068, 133.3747) projected
  line L216 (-22.5068, 133.3747) -> (-22.9168, 133.5446) projected
  line L217 (-22.9168, 133.5446) -> (-23.2688, 133.8147) projected
  line L218 (-23.2688, 133.8147) -> (-23.539, 134.1668) projected
  line L219 (-23.539, 134.1668) -> (-23.7088, 134.5768) projected
  line L220 (-21.4352, 215.2075) -> (-21.4604, 215.6077) projected
  line L221 (-21.4604, 215.6077) -> (-21.4247, 215.8041) projected
  line L222 (-21.4247, 215.8041) -> (-21.42, 215.8311) projected
  line L223 (-21.42, 215.8311) -> (-21.3852, 216.0017) projected
  line L224 (-21.3852, 216.0017) -> (-21.2144, 216.3646) projected
  line L225 (-21.2144, 216.3646) -> (-20.9587, 216.6737) projected
  line L226 (-20.9587, 216.6737) -> (-20.6343, 216.9094) projected
  line L227 (-20.6343, 216.9094) -> (-20.2614, 217.057) projected
  line L228 (-20.2614, 217.057) -> (-19.8635, 217.1073) projected
  line L229 (-19.8635, 217.1073) -> (-19.4656, 217.057) projected
  line L230 (-19.4656, 217.057) -> (-19.0927, 216.9094) projected
  line L231 (-19.0927, 216.9094) -> (-18.7682, 216.6737) projected
  line L232 (-18.7682, 216.6737) -> (-18.5126, 216.3646) projected
  line L233 (-18.5126, 216.3646) -> (-18.3418, 216.0017) projected
  line L234 (-18.3418, 216.0017) -> (-18.2666, 215.6077) projected
  line L235 (-18.2666, 215.6077) -> (-18.2918, 215.2075) projected
  line L236 (-18.2918, 215.2075) -> (-18.4157, 214.8261) projected
  line L237 (-18.4157, 214.8261) -> (-18.6307, 214.4874) projected
  line L238 (-18.6307, 214.4874) -> (-18.923, 214.2129) projected
  line L239 (-18.923, 214.2129) -> (-19.2745, 214.0196) projected
  line L240 (-19.2745, 214.0196) -> (-19.663, 213.9199) projected
  line L241 (-19.663, 213.9199) -> (-20.064, 213.9199) projected
  line L242 (-20.064, 213.9199) -> (-20.4525, 214.0196) projected
  line L243 (-20.4525, 214.0196) -> (-20.8039, 214.2129) projected
  line L244 (-20.8039, 214.2129) -> (-21.0963, 214.4874) projected
  line L245 (-21.0963, 214.4874) -> (-21.3112, 214.8261) projected
  line L246 (-21.3112, 214.8261) -> (-21.4352, 215.2075) projected
  line L247 (-129.6352, 215.2075) -> (-129.6603, 215.6077) projected
  line L248 (-129.6603, 215.6077) -> (-129.5852, 216.0017) projected
  line L249 (-129.5852, 216.0017) -> (-129.4144, 216.3646) projected
  line L250 (-129.4144, 216.3646) -> (-129.1588, 216.6737) projected
  line L251 (-129.1588, 216.6737) -> (-128.8343, 216.9094) projected
  line L252 (-128.8343, 216.9094) -> (-128.4614, 217.057) projected
  line L253 (-128.4614, 217.057) -> (-128.0635, 217.1073) projected
  line L254 (-128.0635, 217.1073) -> (-127.6656, 217.057) projected
  line L255 (-127.6656, 217.057) -> (-127.2927, 216.9094) projected
  line L256 (-127.2927, 216.9094) -> (-126.9682, 216.6737) projected
  line L257 (-126.9682, 216.6737) -> (-126.7125, 216.3646) projected
  line L258 (-126.7125, 216.3646) -> (-126.5418, 216.0017) projected
  line L259 (-126.5418, 216.0017) -> (-126.4666, 215.6077) projected
  line L260 (-126.4666, 215.6077) -> (-126.4918, 215.2075) projected
  line L261 (-126.4918, 215.2075) -> (-126.6158, 214.8261) projected
  line L262 (-126.6158, 214.8261) -> (-126.8307, 214.4874) projected
  line L263 (-126.8307, 214.4874) -> (-127.123, 214.2129) projected
  line L264 (-127.123, 214.2129) -> (-127.4745, 214.0196) projected
  line L265 (-127.4745, 214.0196) -> (-127.863, 213.9199) projected
  line L266 (-127.863, 213.9199) -> (-128.264, 213.9199) projected
  line L267 (-128.264, 213.9199) -> (-128.6525, 214.0196) projected
  line L268 (-128.6525, 214.0196) -> (-129.0039, 214.2129) projected
  line L269 (-129.0039, 214.2129) -> (-129.2963, 214.4874) projected
  line L270 (-129.2963, 214.4874) -> (-129.5112, 214.8261) projected
  line L271 (-129.5112, 214.8261) -> (-129.6352, 215.2075) projected
  line L272 (-129.6352, 1.7901) -> (-129.6603, 2.1903) projected
  line L273 (-129.6603, 2.1903) -> (-129.5852, 2.5843) projected
  line L274 (-129.5852, 2.5843) -> (-129.4144, 2.9472) projected
  line L275 (-129.4144, 2.9472) -> (-129.1588, 3.2563) projected
  line L276 (-129.1588, 3.2563) -> (-128.8343, 3.492) projected
  line L277 (-128.8343, 3.492) -> (-128.4614, 3.6396) projected
  line L278 (-128.4614, 3.6396) -> (-128.0635, 3.6899) projected
  line L279 (-128.0635, 3.6899) -> (-127.6656, 3.6396) projected
  line L280 (-127.6656, 3.6396) -> (-127.2927, 3.492) projected
  line L281 (-127.2927, 3.492) -> (-126.9682, 3.2563) projected
  line L282 (-126.9682, 3.2563) -> (-126.7125, 2.9472) projected
  line L283 (-126.7125, 2.9472) -> (-126.5418, 2.5843) projected
  line L284 (-126.5418, 2.5843) -> (-126.4666, 2.1903) projected
  line L285 (-126.4666, 2.1903) -> (-126.4918, 1.7901) projected
  line L286 (-126.4918, 1.7901) -> (-126.6158, 1.4087) projected
  line L287 (-126.6158, 1.4087) -> (-126.8307, 1.07) projected
  line L288 (-126.8307, 1.07) -> (-127.123, 0.7955) projected
  line L289 (-127.123, 0.7955) -> (-127.4745, 0.6023) projected
  line L290 (-127.4745, 0.6023) -> (-127.863, 0.5025) projected
  line L291 (-127.863, 0.5025) -> (-128.264, 0.5025) projected
  line L292 (-128.264, 0.5025) -> (-128.6525, 0.6023) projected
  line L293 (-128.6525, 0.6023) -> (-129.0039, 0.7955) projected
  line L294 (-129.0039, 0.7955) -> (-129.2963, 1.07) projected
  line L295 (-129.2963, 1.07) -> (-129.5112, 1.4087) projected
  line L296 (-129.5112, 1.4087) -> (-129.6352, 1.7901) projected
  line L297 (-18.0352, 1.7901) -> (-18.0604, 2.1903) projected
  line L298 (-18.0604, 2.1903) -> (-17.9852, 2.5843) projected
  line L299 (-17.9852, 2.5843) -> (-17.8144, 2.9472) projected
  line L300 (-17.8144, 2.9472) -> (-17.5587, 3.2563) projected
  line L301 (-17.5587, 3.2563) -> (-17.2343, 3.492) projected
  line L302 (-17.2343, 3.492) -> (-16.8614, 3.6396) projected
  line L303 (-16.8614, 3.6396) -> (-16.4635, 3.6899) projected
  line L304 (-16.4635, 3.6899) -> (-16.0656, 3.6396) projected
  line L305 (-16.0656, 3.6396) -> (-15.6927, 3.492) projected
  line L306 (-15.6927, 3.492) -> (-15.3682, 3.2563) projected
  line L307 (-15.3682, 3.2563) -> (-15.1126, 2.9472) projected
  line L308 (-15.1126, 2.9472) -> (-14.9418, 2.5843) projected
  line L309 (-14.9418, 2.5843) -> (-14.8667, 2.1903) projected
  line L310 (-14.8667, 2.1903) -> (-14.8918, 1.7901) projected
  line L311 (-14.8918, 1.7901) -> (-15.0158, 1.4087) projected
  line L312 (-15.0158, 1.4087) -> (-15.2307, 1.07) projected
  line L313 (-15.2307, 1.07) -> (-15.523, 0.7955) projected
  line L314 (-15.523, 0.7955) -> (-15.8745, 0.6023) projected
  line L315 (-15.8745, 0.6023) -> (-16.263, 0.5025) projected
  line L316 (-16.263, 0.5025) -> (-16.664, 0.5025) projected
  line L317 (-16.664, 0.5025) -> (-17.0525, 0.6023) projected
  line L318 (-17.0525, 0.6023) -> (-17.4039, 0.7955) projected
  line L319 (-17.4039, 0.7955) -> (-17.6963, 1.07) projected
  line L320 (-17.6963, 1.07) -> (-17.9112, 1.4087) projected
  line L321 (-17.9112, 1.4087) -> (-18.0352, 1.7901) projected
  line L322 (-3.1511, 245.3183) -> (-3.2509, 245.7068) projected
  line L323 (-3.2509, 245.7068) -> (-3.2509, 246.1079) projected
  line L324 (-3.2509, 246.1079) -> (-3.1511, 246.4963) projected
  line L325 (-3.1511, 246.4963) -> (-2.9579, 246.8478) projected
  line L326 (-2.9579, 246.8478) -> (-2.6834, 247.1402) projected
  line L327 (-2.6834, 247.1402) -> (-2.3447, 247.3551) projected
  line L328 (-2.3447, 247.3551) -> (-1.9633, 247.479) projected
  line L329 (-1.9633, 247.479) -> (-1.5631, 247.5042) projected
  line L330 (-1.5631, 247.5042) -> (-1.1691, 247.429) projected
  line L331 (-1.1691, 247.429) -> (-0.8062, 247.2583) projected
  line L332 (-0.8062, 247.2583) -> (-0.4971, 247.0026) projected
  line L333 (-0.4971, 247.0026) -> (-0.2614, 246.6782) projected
  line L334 (-0.2614, 246.6782) -> (-0.1138, 246.3052) projected
  line L335 (-0.1138, 246.3052) -> (-0.0635, 245.9073) projected
  line L336 (-0.0635, 245.9073) -> (-0.1138, 245.5095) projected
  line L337 (-0.1138, 245.5095) -> (-0.2614, 245.1365) projected
  line L338 (-0.2614, 245.1365) -> (-0.4971, 244.812) projected
  line L339 (-0.4971, 244.812) -> (-0.8062, 244.5564) projected
  line L340 (-0.8062, 244.5564) -> (-1.1691, 244.3856) projected
  line L341 (-1.1691, 244.3856) -> (-1.5631, 244.3105) projected
  line L342 (-1.5631, 244.3105) -> (-1.9633, 244.3357) projected
  line L343 (-1.9633, 244.3357) -> (-2.3447, 244.4596) projected
  line L344 (-2.3447, 244.4596) -> (-2.6834, 244.6745) projected
  line L345 (-2.6834, 244.6745) -> (-2.9579, 244.9669) projected
  line L346 (-2.9579, 244.9669) -> (-3.1511, 245.3183) projected
  line L347 (-3.1511, 21.0183) -> (-3.2509, 21.4068) projected
  line L348 (-3.2509, 21.4068) -> (-3.2509, 21.8078) projected
  line L349 (-3.2509, 21.8078) -> (-3.1511, 22.1963) projected
  line L350 (-3.1511, 22.1963) -> (-2.9579, 22.5478) projected
  line L351 (-2.9579, 22.5478) -> (-2.6834, 22.8401) projected
  line L352 (-2.6834, 22.8401) -> (-2.3447, 23.0551) projected
  line L353 (-2.3447, 23.0551) -> (-1.9633, 23.179) projected
  line L354 (-1.9633, 23.179) -> (-1.5631, 23.2042) projected
  line L355 (-1.5631, 23.2042) -> (-1.1691, 23.129) projected
  line L356 (-1.1691, 23.129) -> (-0.8062, 22.9582) projected
  line L357 (-0.8062, 22.9582) -> (-0.4971, 22.7026) projected
  line L358 (-0.4971, 22.7026) -> (-0.2614, 22.3781) projected
  line L359 (-0.2614, 22.3781) -> (-0.1138, 22.0052) projected
  line L360 (-0.1138, 22.0052) -> (-0.0635, 21.6073) projected
  line L361 (-0.0635, 21.6073) -> (-0.1138, 21.2095) projected
  line L362 (-0.1138, 21.2095) -> (-0.2614, 20.8365) projected
  line L363 (-0.2614, 20.8365) -> (-0.4971, 20.5121) projected
  line L364 (-0.4971, 20.5121) -> (-0.8062, 20.2564) projected
  line L365 (-0.8062, 20.2564) -> (-1.1691, 20.0856) projected
  line L366 (-1.1691, 20.0856) -> (-1.5631, 20.0105) projected
  line L367 (-1.5631, 20.0105) -> (-1.9633, 20.0357) projected
  line L368 (-1.9633, 20.0357) -> (-2.3447, 20.1596) projected
  line L369 (-2.3447, 20.1596) -> (-2.6834, 20.3745) projected
  line L370 (-2.6834, 20.3745) -> (-2.9579, 20.6669) projected
  line L371 (-2.9579, 20.6669) -> (-3.1511, 21.0183) projected
  line L372 (2.2365, -1.8101) -> (2.2365, 264.9073) projected
  line L373 (2.2365, 264.9073) -> (-206.7635, 264.9073) projected
  line L374 (-206.7635, 264.9073) -> (-206.7635, -1.8101) projected
  line L375 (-206.7635, -1.8101) -> (2.2365, -1.8101) projected
  circle A0 centre (-1.6635, 245.9073) radius 1.5874
  circle A1 centre (-19.8635, 215.5073) radius 1.5874
  circle A2 centre (-128.0635, 215.5073) radius 1.5874
  circle A3 centre (-128.0635, 2.0899) radius 1.5874
  circle A4 centre (-16.4635, 2.0899) radius 1.5874
  circle A5 centre (-1.6635, 21.6073) radius 1.5874
  circle A6 centre (-57.3517, 134.2073) radius 1.6855
  circle A7 centre (-22.0668, 135.0168) radius 1.6854
  circle A8 centre (-21.7635, 7.9073) radius 1.6855
  circle A9 centre (-88.9635, 7.901) radius 1.6855
  constraints: 30 tangent, 10 centre point
hole "Hole2" at (-1.6635, 3, -245.9073) at (-19.8635, 3, -215.5073) at (-128.0635, 3, -215.5073) at (-57.3517, 3, -134.2073) at (-22.0668, 3, -135.0168) at (-1.6635, 3, -21.6073) at (-21.7635, 3, -7.9073) at (-16.4635, 3, -2.0899) at (-88.9635, 3, -7.901) at (-128.0635, 3, -2.0899) direction (0, -1, 0) diameter 3.4 end through all
sketch "Sketch3" plane through (0, 3, 0) normal (0, 1, 0) x (1, 0, 0)
  point P0 (0, 0)